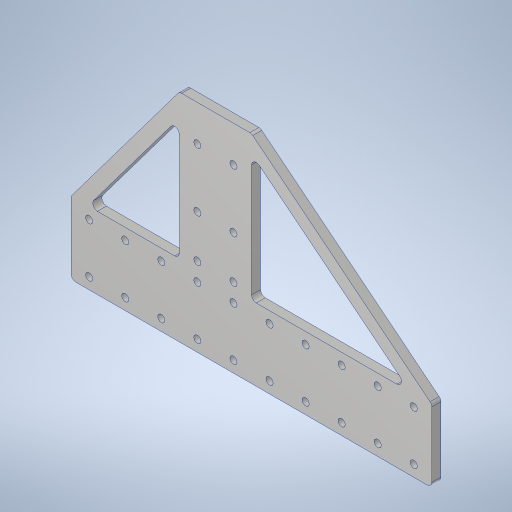
# Autodesk Inventor part: EL2-S-002
Saved by Autodesk Inventor 2023.4 (Build 274418000, 418)
## iProperties
Created: 2025-01-13
Part Number: EL2-S-002
Material: Aluminum 6061
Document SubType Name: Modeling
Designer: mavericks
Density: 2.7 g/cm^3
Appearance: Aluminum - Flat
Author: mavericks
Autodesk Inventor part; units mm, degrees
ref_plane "YZ Plane" through (0, 0, 0) normal (1, 0, 0) x (0, 1, 0)
ref_plane "XZ Plane" through (0, 0, 0) normal (0, 1, 0) x (-1, 0, 0)
ref_plane "XY Plane" through (0, 0, 0) normal (0, 0, 1) x (1, 0, 0)
sketch "Sketch1" plane through (0, 0, 0) normal (0, 0, 1) x (1, 0, 0)
  line L0 (0, 0) -> (50.8, 0) construction
  line L1 (50.8, 0) -> (50.8, 203.2) construction
  line L2 (50.8, 203.2) -> (0, 203.2) construction
  line L3 (0, 203.2) -> (0, 0) construction
  line L4 (-76.2, 0) -> (177.8, 0) construction
  line L5 (177.8, 0) -> (177.8, -50.8) construction
  line L6 (177.8, -50.8) -> (-76.2, -50.8) construction
  line L7 (-76.2, -50.8) -> (-76.2, 0) construction
  line L8 (165.1, -7.9375) -> (165.1, -42.8625) construction
  circle A0 centre (165.1, -7.9375) radius 4.7625 construction
  line L9 (174.625, -3.175) -> (-73.025, -3.175) construction
  line L10 (-73.025, -3.175) -> (-73.025, -47.625) construction
  line L11 (-73.025, -47.625) -> (174.625, -47.625) construction
  line L12 (174.625, -47.625) -> (174.625, -3.175) construction
  circle A1 centre (165.1, -42.8625) radius 4.7625 construction
  line L13 (-76.2, -50.8) -> (-76.2, 0)
  line L14 (-76.2, 0) -> (0, 101.6)
  line L15 (0, 101.6) -> (50.8, 101.6)
  line L16 (50.8, 101.6) -> (177.8, 0)
  line L17 (177.8, 0) -> (177.8, -50.8)
  line L18 (177.8, -50.8) -> (-76.2, -50.8)
  line L19 (50.8, 101.6) -> (50.8, 0) construction
  line L20 (50.8, 0) -> (177.8, 0) construction
  line L21 (0, 101.6) -> (0, 0) construction
  line L22 (0, 0) -> (-76.2, 0) construction
  line L23 (60.325, 9.525) -> (60.325, 81.782) construction
  line L24 (50.8, 89.402) -> (162.5526, 0)
  line L25 (150.6463, 9.525) -> (60.325, 9.525) construction
  line L26 (-64.2937, 0) -> (0, 85.725)
  line L27 (-9.525, 73.025) -> (-9.525, 9.525) construction
  line L28 (-9.525, 9.525) -> (-57.15, 9.525) construction
  line L29 (-64.2937, 0) -> (0, 0)
  line L30 (0, 85.725) -> (0, 0)
  line L31 (50.8, 89.402) -> (50.8, 0)
  line L32 (50.8, 0) -> (162.5526, 0)
  line L33 (-9.525, 9.525) -> (-9.525, 0) construction
  line L34 (12.7, 4.7625) -> (38.1, 4.7625) construction
  line L35 (12.7, 34.925) -> (38.1, 34.925) construction
  point P0 (152.4, -25.4)
  point P1 (165.1, -25.4)
  point P2 (139.7, -42.8625)
  point P3 (139.7, -7.9375)
  point P4 (127, -25.4)
  point P5 (114.3, -42.8625)
  point P6 (114.3, -7.9375)
  point P7 (101.6, -25.4)
  point P8 (88.9, -42.8625)
  point P9 (88.9, -7.9375)
  point P10 (76.2, -25.4)
  point P11 (63.5, -42.8625)
  point P12 (63.5, -7.9375)
  point P13 (50.8, -25.4)
  point P14 (38.1, -42.8625)
  point P15 (38.1, -7.9375)
  point P16 (25.4, -25.4)
  point P17 (12.7, -42.8625)
  point P18 (12.7, -7.9375)
  point P19 (0, -25.4)
  point P20 (-12.7, -42.8625)
  point P21 (-12.7, -7.9375)
  point P22 (-25.4, -25.4)
  point P23 (-38.1, -42.8625)
  point P24 (-38.1, -7.9375)
  point P25 (-50.8, -25.4)
  point P26 (-63.5, -42.8625)
  point P27 (-63.5, -7.9375)
  point P28 (-76.2, -25.4)
  point P29 (12.7, 76.2)
  point P30 (38.1, 76.2)
  point P31 (-9.525, 4.7625)
  point P32 (25.4, 4.7625)
  point P33 (25.4, 34.925)
  dimension "d0" = 50.8
  dimension "d1" = 203.2
  dimension "d2" = 254
  dimension "d3" = 50.8
  dimension "d4" = 127
  dimension "d5" = 12.7
  dimension "d6" = 12.7
  dimension "d7" = 9.525
  dimension "d8" = 3.175
  dimension "d9" = 9.525
  dimension "d12" = 25.4
  dimension "d17" = 25.4
  dimension "d18" = 34.925
  dimension "d19" = 25.4
  dimension "d20" = 12.7
  dimension "d21" = 9.525
  dimension "d22" = 9.525
  dimension "d32" = 85.725
  dimension "d33" = 41.275
  dimension "d35" = 9.525
  dimension "d36" = 9.525
  dimension "d37" = 9.525
  dimension "d38" = 25.4
  constraints: 72 end point, 9 collinear, 9 point on line, 6 horizontal alignment, 6 midpoint, 6 parallel, 5 horizontal, 5 perpendicular, 4 coincident, 4 vertical alignment, 2 centre point, 2 tangent, 1 vertical, 31 other
  measures "d0" distance of L2.end L1.end
  measures "d1" distance of L1.end L0.end
  measures "d2" distance of L5.end L6.end
  measures "d3" distance of L4.end L5.end
  measures "d4" distance of L4.end L0.end
  measures "d5" horizontal distance of point (152.4, -25.4) L8.start
  measures "d6" distance from line of L5 L8.start
  measures "d7" diameter of A0
  measures "d8" distance between parallel lines of L4 L9
  measures "d9" diameter of A1
  measures "d12" distance of L8.end point (139.7, -42.862)
  measures "d17" distance from line of L15 point (12.7, 76.2)
  measures "d18" distance from line of L0 L35.start
  measures "d19" distance of point (12.7, 76.2) point (38.1, 76.2)
  measures "d20" distance from line of L3 point (12.7, 76.2)
  measures "d21" distance between parallel lines of L19 L23
  measures "d22" distance between parallel lines of L22 L28
  measures "d32" distance from line of L6 L35.start
  measures "d33" distance of L35.end point (38.1, 76.2)
  measures "d35" distance between parallel lines of L16 L24
  measures "d36" distance between parallel lines of L14 L26
  measures "d37" distance between parallel lines of L20 L25
  measures "d38" distance of L34.start L34.end
extrude "Extrusion1" add sketch "Sketch1" along normal blind 6.35
hole "Hole1" at (165.1, -7.9375, 0) at (165.1, -42.8625, 0) at (139.7, -42.8625, 0) at (139.7, -7.9375, 0) at (114.3, -42.8625, 0) at (114.3, -7.9375, 0) at (88.9, -42.8625, 0) at (88.9, -7.9375, 0) at (63.5, -42.8625, 0) at (63.5, -7.9375, 0) at (38.1, -42.8625, 0) at (38.1, -7.9375, 0) at (12.7, -42.8625, 0) at (12.7, -7.9375, 0) at (-12.7, -42.8625, 0) at (-12.7, -7.9375, 0) at (-38.1, -42.8625, 0) at (-38.1, -7.9375, 0) at (-63.5, -42.8625, 0) at (-63.5, -7.9375, 0) at (12.7, 76.2, 0) at (38.1, 76.2, 0) at (38.1, 34.925, 0) at (12.7, 34.925, 0) at (12.7, 4.7625, 0) at (38.1, 4.7625, 0) direction (0, 0, 1) diameter 5.1054 end through all clearance for "Flat Head Machine Screw (82)" size "#10" standard "Ansi Unified Screw Threads"
fillet "Fillet1" radius 3.302 12 edges at (50.8, 101.6, 3.175) (0, 101.6, 3.175) (177.8, 0, 3.175) (-76.2, 0, 3.175) (-76.2, -50.8, 3.175) (177.8, -50.8, 3.175) (50.8, 0, 3.175) (50.8, 89.402, 3.175) (0, 85.725, 3.175) (0, 0, 3.175) (-64.2937, 0, 3.175) (162.5526, 0, 3.175)
body "Solid1"
